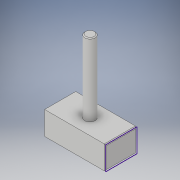
# Autodesk Inventor part: Mjolnir
Saved by Autodesk Inventor 2017 (Build 210142000, 142)
## iProperties
Created: 2016-12-22
Part Number: Mjolnir
Material: Generic
Document SubType Name: Modeling
Designer: theoren75306
Density: 1 g/cm^3
Appearance: Default
Author: theoren75306
Autodesk Inventor part; units mm, degrees
ref_plane "YZ Plane" through (0, 0, 0) normal (1, 0, 0) x (0, 1, 0)
ref_plane "XZ Plane" through (0, 0, 0) normal (0, 1, 0) x (-1, 0, 0)
ref_plane "XY Plane" through (0, 0, 0) normal (0, 0, 1) x (1, 0, 0)
sketch "Sketch1" plane through (0, 0, 0) normal (0, 1, 0) x (-1, 0, 0)
  line L0 (0, 0) -> (304.8, 0)
  line L1 (304.8, 0) -> (304.8, -152.4)
  line L2 (304.8, -152.4) -> (0, -152.4)
  line L3 (0, -152.4) -> (0, 0)
  dimension "d0" = 304.8
  dimension "d1" = 152.4
  constraints: 8 end point, 2 parallel, 1 horizontal, 1 perpendicular
  measures "d0" distance of L1.end L2.end
  measures "d1" distance of L0.end L1.end
extrude "Extrusion1" add sketch "Sketch1" along normal blind 114.3
sketch "Sketch2" plane through (0, 114.3, 0) normal (0, 1, 0) x (1, 0, 0)
  circle A0 centre (-152.4, 76.2) radius 25.4
  line L0 (0, 0) -> (0, 152.4) projected
  line L1 (0, 152.4) -> (-304.8, 152.4) projected
  dimension "d4" = 152.4
  dimension "d5" = 76.2
  dimension "d6" = 50.8
  constraints: 1 centre point
  measures "d4" distance from line of L0 A0.centre
  measures "d5" distance from line of L1 A0.centre
  measures "d6" diameter of A0
extrude "Extrusion2" add sketch "Sketch2" along normal blind 355.6
sketch "Sketch3" plane through (0, 0, 0) normal (1, 0, 0) x (0, 0, -1)
  line L0 (152.4, 0) -> (152.4, 114.3) projected
  line L1 (0, 0) -> (152.4, 0)
  line L2 (152.4, 0) -> (152.4, 114.3)
  line L3 (152.4, 114.3) -> (0, 114.3)
  line L4 (0, 114.3) -> (0, 0)
  constraints: 8 end point, 2 parallel, 1 horizontal, 1 perpendicular
chamfer "Chamfer1" distance 6.35 angle 45 1 edges at (0, 114.3, -76.2)
chamfer "Chamfer2" distance 6.35 angle 45 1 edges at (0, 53.975, 0)
chamfer "Chamfer3" distance 6.35 angle 45 1 edges at (0, 0, -79.375)
chamfer "Chamfer4" distance 6.35 angle 45 1 edges at (0, 57.15, -152.4)
chamfer "Chamfer5" distance 6.35 angle 45 4 edges at (-304.8, 114.3, -76.2) (-304.8, 57.15, -152.4) (-304.8, 57.15, 0) (-304.8, 0, -76.2)
chamfer "Chamfer6" distance 4.445 angle 45 1 edges at (-177.8, 469.9, -76.2)
sketch "Sketch4" plane through (0, 0, 0) normal (0, -1, 0) x (1, 0, 0)
  circle A0 centre (-152.4, -76.2) radius 25.4 projected
  circle A1 centre (-152.4, -76.2) radius 25.4
  point P0 (0, 0)
  constraints: 1 centre point, 1 coincident
extrude "Extrusion3" add sketch "Sketch4" along normal blind 6.35
body "Solid1"
